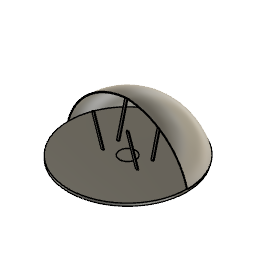
Drone-Station (Autodesk Fusion 360 archive; units mm, degrees)
design "Drone-Station"
part number: 2026-08-28-14-55-35-797
Autodesk Fusion 360 part; units mm, degrees
sketch "Sketch1" plane through (0, 0, 0) normal (0, 0, 1) x (1, 0, 0)
  circle A0 centre (0, 0) radius 1100
  circle A1 centre (0, 0) radius 150
  dimension "d1" = 2200
  dimension "d2" = 300
  constraint coincident A0.centre A1.centre
  constraint concentric A0 A1
  measures "d1" diameter of A0
  measures "d2" diameter of A1
extrude "Extrude1" add sketch "Sketch1" against normal blind 50 makes body 1
extrude "Extrude2" add sketch "Sketch1" against normal blind 40 separate body contours A1 makes body 2
sketch "Sketch2" plane through (0, 0, 0) normal (0, 1, 0) x (1, 0, 0)
  arc A0 (-1100, 0) -> (0, -900) centre (73.6505, 312.2394) ccw
  arc A1 (-1113.5882, -6.3529) -> (0, -914.7946) centre (73.6505, 312.2394) ccw
  line L0 (-1100, 0) -> (1100, 0)
  line L1 (1100, 0) -> (1113.5882, 0)
  line L2 (1113.5882, 0) -> (1113.5882, -6.3529)
  line L3 (-1100, 0) -> (-1113.5918, 0)
  line L4 (-1113.5918, 0) -> (-1113.5882, -6.3529)
  line L5 (0, 0) -> (0, -914.7946)
  constraint horizontal L0
  constraint parallel L0 L1
  constraint perpendicular L0 L2
  constraint perpendicular L2 L3
  constraint coincident L5.start origin
  constraint perpendicular L0 L5
  constraint concentric A0 A1
  constraint coincident L5 A0.end
revolve "Revolve1" add sketch "Sketch2" angle 180 about axis through (0, 0, 0) along (0, 0, -1) separate body contours A0 A1 L3 L4 L5 makes body 3
mirror "Mirror1" about plane through (0, 0, 0) normal (0, 1, 0) of bodies 3 makes body 4
sketch "Sketch3" plane through (0, 0, 0) normal (1, 0, 0) x (0, 1, 0)
  line L0 (-150.673, 2.5519) -> (-329.0417, 705.3877)
  line L1 (150.673, 2.5519) -> (329.0417, 705.3877)
  line L2 (-136.1339, 6.2417) -> (-314.5026, 709.0775)
  line L3 (-314.5026, 709.0775) -> (-329, 709.0775)
  line L4 (-329, 709.0775) -> (-329.0417, 705.3877)
  line L5 (136.1339, 6.2417) -> (314.5026, 709.0775)
  line L6 (314.5026, 709.0775) -> (329.0417, 709.0775)
  line L7 (329.0417, 709.0775) -> (329.0417, 705.3877)
  line L8 (-150.673, 2.5519) -> (-150.673, 0)
  line L9 (-150.673, 0) -> (-136.1339, 0)
  line L10 (-136.1339, 0) -> (-136.1339, 6.2417)
  line L11 (150.673, 2.5519) -> (150.673, 0)
  line L12 (150.673, 0) -> (136.1339, 0)
  line L13 (136.1339, 0) -> (136.1339, 6.2417)
  dimension "d13" = 15
  dimension "d14" = -15
  constraint horizontal L3
  constraint horizontal L6
  constraint perpendicular L6 L7
  constraint vertical L8
  constraint perpendicular L8 L9
  constraint perpendicular L9 L10
  constraint parallel L10 L11
  constraint perpendicular L11 L12
  constraint perpendicular L12 L13
extrude "Extrude3" add sketch "Sketch3" along normal blind 40 separate body contours L0 L2 L3 L4 L8 L9 L10 makes body 5
extrude "Extrude4" add sketch "Sketch3" along normal blind 40 separate body contours L1 L5 L6 L7 L11 L12 L13 makes body 6
move_body "Move1" bodies 5 to x (1, 0, 0) y (0, 1, 0) z (0, 0, 1) at (300, 0, 0)
move_body "Move2" bodies 6 to x (1, 0, 0) y (0, 1, 0) z (0, 0, 1) at (300, 0, 0)
mirror "Mirror2" about plane through (0, 0, 0) normal (1, 0, 0) of bodies 5 makes body 7
mirror "Mirror3" about plane through (0, 0, 0) normal (1, 0, 0) of bodies 6 makes body 8
hidden bodies 4
